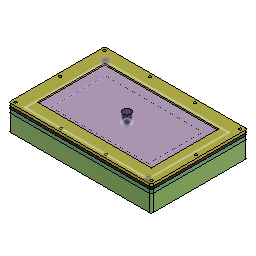
e-ink-photo-frame (Autodesk Fusion 360 design; units mm, degrees)
Autodesk Fusion 360 part; units mm, degrees
(part 1 of 2)
sketch "Sketch1" plane through (0, 0, 0) normal (0, 0, 1) x (1, 0, 0) in component "display-frame"
  line L0 (86, 56) -> (-86, 56)
  line L1 (-86, 56) -> (-86, -56)
  line L2 (-86, -56) -> (86, -56)
  line L3 (86, -56) -> (86, 56)
  line L4 (86, 56) -> (-86, -56) construction
  line L5 (-86, 56) -> (86, -56) construction
  line L6 (15, -65.5) -> (15, -56)
  line L7 (15, -56) -> (-15, -56)
  line L8 (-15, -56) -> (-15, -65.5)
  line L9 (-68, 38) -> (-68, -38)
  line L10 (-68, -38) -> (68, -38)
  line L11 (68, -38) -> (68, 38)
  line L12 (68, 38) -> (-68, 38)
  line L13 (-15, -58.5) -> (15, -58.5)
  line L14 (-15, -59.5) -> (15, -59.5)
  line L15 (80, 49) -> (-80, 49) construction
  line L16 (-80, 49) -> (-80, -46) construction
  line L17 (-80, -46) -> (80, -46) construction
  line L18 (80, -46) -> (80, 49) construction
  line L19 (80, 49) -> (-80, -46) construction
  line L20 (-80, 49) -> (80, -46) construction
  line L21 (-99.5, 68.5) -> (-99.5, -65.5)
  line L22 (-99.5, -65.5) -> (99.5, -65.5)
  line L23 (99.5, -65.5) -> (99.5, 68.5)
  line L24 (99.5, 68.5) -> (-99.5, 68.5)
  point P0 (0, -56)
  point P1 (0, -56)
  point P2 (0, 1.5)
  dimension "d1" = 112
  dimension "d2" = 172
  dimension "d6" = 30
  dimension "d8" = 2.5
  dimension "d30" = 1
  dimension "d86" = -18
  dimension "d91" = 30
  dimension "d93" = 160
  dimension "d94" = 95
  dimension "d96" = 19.5
  dimension "d97" = 9.5
  dimension "d101" = 10
  constraint horizontal L0
  constraint perpendicular L0 L1
  constraint parallel L0 L2
  constraint parallel L1 L3
  constraint coincident L4 origin
  constraint coincident L5 origin
  constraint vertical L6
  constraint horizontal L7
  constraint vertical L8
  constraint coincident L2 L6.end
  constraint midpoint L2 P1
  constraint midpoint L7 P1
  constraint coincident P1 P0
  constraint coincident L8 L13.start
  constraint coincident L6 L13.end
  constraint perpendicular L6 L13
  constraint coincident L8 L14.start
  constraint coincident L6 L14.end
  constraint perpendicular L6 L14
  constraint horizontal L15
  constraint perpendicular L15 L16
  constraint parallel L15 L17
  constraint parallel L16 L18
  constraint coincident L19 P2
  constraint coincident L20 P2
  constraint vertical origin P2
  constraint coincident L8.end L22
  constraint coincident L6.start L22
  measures "d1" distance of L0.end L1.end
  measures "d2" distance of L0.start L0.end
  measures "d6" distance of L6 L8
  measures "d8" distance of L7 L13
  measures "d30" distance of L13 L14
  measures "d91" distance of L14.start L14.end
  measures "d93" distance of L15.start L15.end
  measures "d94" distance of L15.end L16.end
  measures "d97" distance of L2 L22
  measures "d101" distance of L2 L17
extrude "Extrude4" add sketch "Sketch1" along normal blind 0.5 contours L0 L1 L2 L3 L7 | L0 L1 L2 L3 L6 L8 L21 L22 L23 L24 | L2 L6 L7 L8 L13 | L6 L8 L14 L22 makes body 1 in component "display-frame"
extrude "Extrude5" add sketch "Sketch1" along normal blind 3.5 contours L0 L1 L2 L3 L6 L8 L21 L22 L23 L24 | L6 L8 L14 L22 bodies 1 in component "display-frame"
extrude "Extrude6" add sketch "Sketch1" along normal blind 2.5 contours L2 L6 L7 L8 L13 bodies 1 in component "display-frame"
fillet "Fillet3" radius 2.5 1 edges at (0, -58.5, 2.5) on bodies 1 in component "display-frame"
fillet "Fillet4" radius 2.5 4 edges at (-99.5, -65.5, 1.75) (-99.5, 68.5, 1.75) (99.5, 68.5, 1.75) (99.5, -65.5, 1.75) on bodies 1 in component "display-frame"
sketch "Sketch4" plane through (0, 0, 3.5) normal (0, 0, 1) x (-1, 0, 0) in component "display-frame"
  line L0 (-15, 59.5) -> (15, 59.5)
  line L1 (15, 59.5) -> (15, 56)
  line L2 (15, 56) -> (86, 56)
  line L3 (86, 56) -> (86, -56)
  line L4 (86, -56) -> (-86, -56)
  line L5 (-86, -56) -> (-86, 56)
  line L6 (-86, 56) -> (-15, 56)
  line L7 (-15, 56) -> (-15, 59.5)
  arc A0 (-97, 65.5) -> (-99.5, 63) centre (-97, 63) ccw
  line L8 (-99.5, 63) -> (-99.5, -66)
  arc A1 (-99.5, -66) -> (-97, -68.5) centre (-97, -66) ccw
  line L9 (-97, -68.5) -> (97, -68.5)
  arc A2 (97, -68.5) -> (99.5, -66) centre (97, -66) ccw
  line L10 (99.5, -66) -> (99.5, 63)
  arc A3 (99.5, 63) -> (97, 65.5) centre (97, 63) ccw
  line L11 (97, 65.5) -> (-97, 65.5)
  line L12 (99.5, -63.75) -> (-99.5, -63.75) construction
  line L13 (-94.75, -68.5) -> (-94.75, 65.5) construction
  line L14 (99.5, 60.75) -> (-99.5, 60.75) construction
  line L15 (94.75, 65.5) -> (94.75, -68.5) construction
  circle A4 centre (94.75, 60.75) radius 1.75
  circle A5 centre (94.75, -63.75) radius 1.75
  circle A6 centre (31.5833, -63.75) radius 1.75
  circle A7 centre (-31.5833, -63.75) radius 1.75
  circle A8 centre (-94.75, -63.75) radius 1.75
  circle A9 centre (-94.75, 60.75) radius 1.75
  circle A10 centre (-94.75, -1.5) radius 1.75
  circle A11 centre (31.5833, 60.75) radius 1.75
  circle A12 centre (-31.5833, 60.75) radius 1.75
  circle A13 centre (94.75, -1.5) radius 1.75
  dimension "d117" = 9.5
  dimension "d118" = 4.75
  dimension "d119" = 4.75
  dimension "d120" = 4.75
  dimension "d121" = 4.75
  dimension "d122" = 3.5
  dimension "d123" = 189.5
  dimension "d124" = 63.1667
  dimension "d125" = 63.1667
  constraint coincident L10 L12.start
  constraint coincident L8 L12.end
  constraint perpendicular L8 L12
  constraint coincident L9 L13.start
  constraint coincident L11 L13.end
  constraint perpendicular L11 L13
  constraint coincident L10 L14.start
  constraint coincident L8 L14.end
  constraint perpendicular L8 L14
  constraint coincident L11 L15.start
  constraint coincident L9 L15.end
  constraint perpendicular L9 L15
  constraint coincident L15 A4.centre
  constraint coincident L14 A4.centre
  constraint coincident L15 A5.centre
  constraint coincident L12 A5.centre
  constraint coincident L12 A6.centre
  constraint coincident L12 A7.centre
  constraint coincident L13 A8.centre
  constraint coincident L12 A8.centre
  constraint coincident L13 A9.centre
  constraint coincident L14 A9.centre
  constraint midpoint L13 A10.centre
  constraint coincident L14 A11.centre
  constraint coincident L14 A12.centre
  constraint midpoint L15 A13.centre
  constraint equal A5 A6
  constraint equal A6 A7
  constraint equal A7 A8
  constraint equal A8 A10
  constraint equal A9 A10
  constraint equal A9 A12
  constraint equal A11 A12
  constraint equal A4 A11
  constraint equal A4 A13
  constraint vertical A6.centre A11.centre
  constraint vertical A7.centre A12.centre
  measures "d117" distance of L2 L11
  measures "d118" distance of L11 L14
  measures "d119" distance of L10 L15
  measures "d120" distance of L9 L12
  measures "d121" distance of L8 L13
  measures "d122" diameter of A4
  measures "d123" distance of A5.centre A8.centre
  measures "d124" distance of A5.centre A6.centre
  measures "d125" distance of A7.centre A8.centre
extrude "Extrude9" cut sketch "Sketch4" against normal blind 35 contours A4 | A5 | A6 | A7 | A8 | A9 | A10 | A11 | A12 | A13 bodies 1 in component "display-frame"
sketch "Sketch1 (2)" plane through (0, 0, 0) normal (0, 0, -1) x (1, 0, 0) in component "controller-frame"
  circle A0 centre (31.5833, 60.75) radius 1.75
  circle A1 centre (31.5833, -63.75) radius 1.75
  circle A2 centre (-94.75, -1.5) radius 1.75
  circle A3 centre (94.75, -63.75) radius 1.75
  circle A4 centre (-31.5833, 60.75) radius 1.75
  circle A5 centre (94.75, 60.75) radius 1.75
  circle A6 centre (-31.5833, -63.75) radius 1.75
  circle A7 centre (-94.75, -63.75) radius 1.75
  circle A8 centre (94.75, -1.5) radius 1.75
  circle A9 centre (-94.75, 60.75) radius 1.75
  arc A10 (99.5, 63) -> (97, 65.5) centre (97, 63) ccw
  line L0 (97, 65.5) -> (-97, 65.5)
  arc A11 (-97, 65.5) -> (-99.5, 63) centre (-97, 63) ccw
  line L1 (-99.5, 63) -> (-99.5, -66)
  arc A12 (-99.5, -66) -> (-97, -68.5) centre (-97, -66) ccw
  line L2 (-97, -68.5) -> (97, -68.5)
  arc A13 (97, -68.5) -> (99.5, -66) centre (97, -66) ccw
  line L3 (99.5, -66) -> (99.5, 63)
  line L4 (15, 58.5) -> (-15, 58.5)
  line L5 (-15, 58.5) -> (-15, 59.5)
  line L6 (-15, 59.5) -> (15, 59.5)
  line L7 (15, 59.5) -> (15, 58.5)
  line L8 (68, -38) -> (-68, -38)
  line L9 (-68, -38) -> (-68, 38)
  line L10 (-68, 38) -> (68, 38)
  line L11 (68, 38) -> (68, -38)
  line L12 (-86, 56) -> (86, 56)
  line L13 (86, 56) -> (86, -56)
  line L14 (86, -56) -> (-86, -56)
  line L15 (-86, -56) -> (-86, 56)
  line L16 (-68, -38) -> (68, -38)
  line L17 (68, -38) -> (68, 38)
  line L18 (68, 38) -> (-68, 38)
  line L19 (-68, 38) -> (-68, -38)
  line L20 (-15, 56) -> (-15, 58.5)
  line L21 (-15, 58.5) -> (15, 58.5)
  line L22 (15, 58.5) -> (15, 56)
  line L23 (15, 56) -> (-15, 56)
extrude "Extrude2" add sketch "Sketch1 (2)" along normal blind 2.5 separate body contours A10 L0 A11 L1 A12 L2 A13 L3 | L4 L12 L20 L21 L22 L23 | L12 L13 L14 L15 L23 | L8 L9 L10 L11 L16 L17 L18 L19 makes body 2 in component "controller-frame"
sketch "Sketch2" plane through (0, 0, -2.5) normal (0, 0, -1) x (1, 0, 0) in component "controller-frame"
  line L0 (-15, 58.5) -> (-15, 59.5)
  line L1 (15, 59.5) -> (15, 58.5)
  line L2 (15, 58.5) -> (-15, 58.5)
  line L3 (-86, 56) -> (86, 56)
  line L4 (86, 56) -> (86, -56)
  line L5 (86, -56) -> (-86, -56)
  line L6 (-86, -56) -> (-86, 56)
  line L7 (-68, -38) -> (68, -38)
  line L8 (68, -38) -> (68, 38)
  line L9 (68, 38) -> (-68, 38)
  line L10 (-68, 38) -> (-68, -38)
  line L11 (-29, -12) -> (29, -12) construction
  line L12 (29, -12) -> (29, -35) construction
  line L13 (29, -35) -> (-29, -35) construction
  line L14 (-29, -35) -> (-29, -12) construction
  line L15 (-29, -12) -> (29, -35) construction
  line L16 (29, -12) -> (-29, -35) construction
  line L17 (-21.25, 52) -> (21.25, 52) construction
  line L18 (21.25, 52) -> (21.25, 33.5) construction
  line L19 (21.25, 33.5) -> (-21.25, 33.5) construction
  line L20 (-21.25, 33.5) -> (-21.25, 52) construction
  line L21 (-21.25, 52) -> (21.25, 33.5) construction
  line L22 (21.25, 52) -> (-21.25, 33.5) construction
  circle A0 centre (29, -35) radius 1.75
  circle A1 centre (-29, -35) radius 1.75
  circle A2 centre (-29, -12) radius 1.75
  circle A3 centre (29, -12) radius 1.75
  circle A4 centre (29, -35) radius 3
  circle A5 centre (-29, -35) radius 3
  circle A6 centre (-29, -12) radius 3
  circle A7 centre (29, -12) radius 3
  circle A8 centre (18.75, 36) radius 2.5 construction
  circle A9 centre (18.75, 36) radius 1.75
  circle A10 centre (-18.75, 36) radius 2.5 construction
  circle A11 centre (-18.75, 36) radius 1.75
  circle A12 centre (18.75, 49.5) radius 2.5 construction
  circle A13 centre (18.75, 49.5) radius 1
  circle A14 centre (-18.75, 49.5) radius 2.5 construction
  circle A15 centre (-18.75, 49.5) radius 1
  line L23 (-15, 59.5) -> (15, 59.5)
  circle A16 centre (-31.5833, 60.75) radius 1.75
  circle A17 centre (94.75, -1.5) radius 1.75
  circle A18 centre (31.5833, 60.75) radius 1.75
  circle A19 centre (31.5833, -63.75) radius 1.75
  circle A20 centre (-94.75, -1.5) radius 1.75
  circle A21 centre (94.75, -63.75) radius 1.75
  circle A22 centre (-94.75, 60.75) radius 1.75
  circle A23 centre (-94.75, -63.75) radius 1.75
  circle A24 centre (-31.5833, -63.75) radius 1.75
  circle A25 centre (94.75, 60.75) radius 1.75
  line L24 (99.5, -66) -> (99.5, 63)
  arc A26 (99.5, 63) -> (97, 65.5) centre (97, 63) ccw
  line L25 (97, 65.5) -> (-97, 65.5)
  arc A27 (-97, 65.5) -> (-99.5, 63) centre (-97, 63) ccw
  line L26 (-99.5, 63) -> (-99.5, -66)
  arc A28 (-99.5, -66) -> (-97, -68.5) centre (-97, -66) ccw
  line L27 (-97, -68.5) -> (97, -68.5)
  arc A29 (97, -68.5) -> (99.5, -66) centre (97, -66) ccw
  line L28 (-15, 56) -> (-15, 58.5)
  line L29 (-15, 58.5) -> (15, 58.5)
  line L30 (15, 58.5) -> (15, 56)
  line L31 (15, 56) -> (-15, 56)
  point P0 (0, -23.5)
  point P1 (0, 42.75)
  dimension "d134" = 23
  dimension "d135" = 58
  dimension "d136" = 3.5
  dimension "d137" = 6
  dimension "d140" = 5
  dimension "d141" = 3.5
  dimension "d142" = 2
  dimension "d143" = 7.5
  dimension "d234" = 13.5
  dimension "d235" = 37.5
  constraint horizontal L11
  constraint perpendicular L11 L12
  constraint parallel L11 L13
  constraint parallel L12 L14
  constraint coincident L15 P0
  constraint coincident L16 P0
  constraint horizontal L17
  constraint perpendicular L17 L18
  constraint parallel L17 L19
  constraint parallel L18 L20
  constraint coincident L21 P1
  constraint coincident L22 P1
  constraint vertical origin P0
  constraint vertical origin P1
  constraint coincident L12.end L13.start
  constraint coincident L13.end L14.start
  constraint coincident L11.start L14.end
  constraint coincident L11.end L12.start
  constraint equal A2 A3
  constraint equal A1 A2
  constraint equal A0 A1
  constraint concentric A2 A6
  constraint concentric A3 A7
  constraint equal A6 A7
  constraint equal A5 A6
  constraint equal A4 A5
  constraint tangent L7 A4
  constraint concentric A8 A9
  constraint tangent L19 A8
  constraint tangent L18 A8
  constraint concentric A10 A11
  constraint concentric A12 A13
  constraint concentric A14 A15
  constraint equal A13 A15
  constraint equal A9 A11
  constraint equal A10 A14
  constraint equal A12 A14
  constraint equal A8 A12
  constraint tangent L19 A10
  constraint tangent L20 A10
  constraint tangent L17 A12
  constraint tangent L18 A12
  constraint tangent L20 A14
  constraint tangent L17 A14
  measures "d134" distance of L11.end L12.end
  measures "d135" distance of L11.start L11.end
  measures "d136" diameter of A0
  measures "d137" diameter of A4
  measures "d140" diameter of A8
  measures "d141" diameter of A9
  measures "d142" diameter of A13
  measures "d143" distance of L0.end L17
  measures "d234" distance of A8.centre A12.centre
  measures "d235" distance of A8.centre A10.centre
extrude "Extrude4'" add sketch "Sketch2" along normal blind 2.5 contours A5 | A4 | A6 | A7 | A13 | A15 | L24 A26 L25 A27 L26 A28 L27 A29 bodies 2 in component "controller-frame"
extrude "Extrude5'" cut sketch "Sketch2" against normal blind 27 contours A0 | A1 | A2 | A3 | A9 | A11 bodies 2 in component "controller-frame"
fillet "Fillet1" radius 2.5 4 edges at (26.203, 33.9152, -2.5) (-31.797, 33.9152, -2.5) (-31.797, 10.9152, -2.5) (26.203, 10.9152, -2.5) on bodies 2 in component "controller-frame"
fillet "Fillet2" radius 2.5 4 edges at (86, 56, -3.75) (86, -56, -3.75) (-86, -56, -3.75) (-86, 56, -3.75) on bodies 2 in component "controller-frame"
fillet "Fillet3'" radius 2.5 1 edges at (0, -58.5, -2.5) on bodies 2 in component "controller-frame"
sketch "Sketch1 (3)" plane through (0, 0, -5) normal (0, 0, -1) x (1, 0, 0) in component "backing-frame"
  circle A0 centre (-94.75, -63.75) radius 1.75
  line L0 (15, 59.5) -> (15, 56)
  line L1 (15, 56) -> (83.5, 56)
  arc A1 (86, 53.5) -> (83.5, 56) centre (83.5, 53.5) ccw
  line L2 (86, 53.5) -> (86, -53.5)
  arc A2 (83.5, -56) -> (86, -53.5) centre (83.5, -53.5) ccw
  line L3 (83.5, -56) -> (-83.5, -56)
  arc A3 (-86, -53.5) -> (-83.5, -56) centre (-83.5, -53.5) ccw
  line L4 (-86, -53.5) -> (-86, 53.5)
  arc A4 (-83.5, 56) -> (-86, 53.5) centre (-83.5, 53.5) ccw
  line L5 (-83.5, 56) -> (-15, 56)
  line L6 (-15, 56) -> (-15, 59.5)
  line L7 (-15, 59.5) -> (15, 59.5)
  circle A5 centre (-94.75, -1.5) radius 1.75
  circle A6 centre (-31.5833, -63.75) radius 1.75
  circle A7 centre (94.75, 60.75) radius 1.75
  circle A8 centre (31.5833, 60.75) radius 1.75
  circle A9 centre (-31.5833, 60.75) radius 1.75
  circle A10 centre (-94.75, 60.75) radius 1.75
  circle A11 centre (94.75, -63.75) radius 1.75
  circle A12 centre (94.75, -1.5) radius 1.75
  circle A13 centre (31.5833, -63.75) radius 1.75
  arc A14 (97, -68.5) -> (99.5, -66) centre (97, -66) ccw
  line L8 (99.5, -66) -> (99.5, 63)
  arc A15 (99.5, 63) -> (97, 65.5) centre (97, 63) ccw
  line L9 (97, 65.5) -> (-97, 65.5)
  arc A16 (-97, 65.5) -> (-99.5, 63) centre (-97, 63) ccw
  line L10 (-99.5, 63) -> (-99.5, -66)
  arc A17 (-99.5, -66) -> (-97, -68.5) centre (-97, -66) ccw
  line L11 (-97, -68.5) -> (97, -68.5)
  line L12 (15, 58.5) -> (15, 56)
  line L13 (15, 58.5) -> (-15, 58.5)
  line L14 (-15, 56) -> (-15, 58.5)
  line L15 (-15, 56) -> (15, 56)
extrude "Extrude2'" add sketch "Sketch1 (3)" along normal blind 3 separate body contours L0 L6 L7 L13 | L0 L6 L12 L13 L14 L15 | A14 L8 A15 L9 A16 L10 A17 L11 makes body 3 in component "backing-frame"
sketch "Sketch3" plane through (0, 0, -8) normal (0, 0, -1) x (1, 0, 0) in component "backing-frame"
  circle A0 centre (31.5833, -63.75) radius 1.75
  circle A1 centre (94.75, -1.5) radius 1.75
  circle A2 centre (94.75, -63.75) radius 1.75
  circle A3 centre (31.5833, 60.75) radius 1.75
  line L0 (-83.5, 56) -> (83.5, 56)
  arc A4 (86, 53.5) -> (83.5, 56) centre (83.5, 53.5) ccw
  line L1 (86, 53.5) -> (86, -53.5)
  arc A5 (83.5, -56) -> (86, -53.5) centre (83.5, -53.5) ccw
  line L2 (83.5, -56) -> (-83.5, -56)
  line L3 (-86, -53.5) -> (-86, 53.5)
  circle A6 centre (94.75, 60.75) radius 1.75
  line L4 (-97, -68.5) -> (97, -68.5)
  arc A7 (97, -68.5) -> (99.5, -66) centre (97, -66) ccw
  line L5 (99.5, -66) -> (99.5, 63)
  arc A8 (99.5, 63) -> (97, 65.5) centre (97, 63) ccw
  line L6 (97, 65.5) -> (-97, 65.5)
  line L7 (-99.5, 63) -> (-99.5, -66)
  line L8 (94.75, -63.75) -> (83.5, -53.5) construction
  line L9 (94.75, 60.75) -> (83.5, 53.5) construction
  line L10 (94.75, -1.5) -> (86, -1.5) construction
  line L11 (31.5833, -63.75) -> (31.5833, -56) construction
  line L12 (31.5833, 60.75) -> (31.5833, 56) construction
  line L13 (91.65, -3.2898) -> (94.75, -5.0796)
  line L14 (94.75, -5.0796) -> (97.85, -3.2898)
  line L15 (97.85, -3.2898) -> (97.85, 0.2898)
  line L16 (97.85, 0.2898) -> (94.75, 2.0796)
  line L17 (94.75, 2.0796) -> (91.65, 0.2898)
  line L18 (91.65, 0.2898) -> (91.65, -3.2898)
  line L19 (94.75, -5.0796) -> (86, -5.0796)
  line L20 (94.75, 2.0796) -> (86, 2.0796)
  line L21 (81.641, -56) -> (93.9852, -67.2469)
  line L22 (93.9852, -67.2469) -> (97.396, -66.1608)
  line L23 (97.396, -66.1608) -> (98.1608, -62.6639)
  line L24 (98.1608, -62.6639) -> (86, -51.584)
  line L25 (95.5148, -60.2531) -> (92.104, -61.3392)
  line L26 (92.104, -61.3392) -> (91.3392, -64.8361)
  line L27 (86, 51.4231) -> (97.9337, 59.1138)
  line L28 (97.9337, 59.1138) -> (97.7589, 62.6891)
  line L29 (97.7589, 62.6891) -> (94.5752, 64.3253)
  line L30 (94.5752, 64.3253) -> (81.6566, 56)
  line L31 (91.5663, 62.3862) -> (91.7411, 58.8109)
  line L32 (91.7411, 58.8109) -> (94.9248, 57.1747)
  line L33 (29.7935, -60.65) -> (28.0038, -63.75)
  line L34 (28.0038, -63.75) -> (29.7935, -66.85)
  line L35 (29.7935, -66.85) -> (33.3731, -66.85)
  line L36 (33.3731, -66.85) -> (35.1629, -63.75)
  line L37 (35.1629, -63.75) -> (33.3731, -60.65)
  line L38 (33.3731, -60.65) -> (29.7935, -60.65)
  line L39 (28.0038, -63.75) -> (28.0038, -56)
  line L40 (35.1629, -63.75) -> (35.1629, -56)
  line L41 (33.3731, 57.65) -> (35.1629, 60.75)
  line L42 (35.1629, 60.75) -> (33.3731, 63.85)
  line L43 (33.3731, 63.85) -> (29.7935, 63.85)
  line L44 (29.7935, 63.85) -> (28.0038, 60.75)
  line L45 (28.0038, 60.75) -> (29.7935, 57.65)
  line L46 (29.7935, 57.65) -> (33.3731, 57.65)
  line L47 (28.0038, 60.75) -> (28.0038, 56)
  line L48 (35.1629, 60.75) -> (35.1629, 56)
  line L49 (0, -68.5) -> (0, 65.5) construction
  line L50 (-29.7935, 63.85) -> (-28.0038, 60.75)
  line L51 (-33.3731, 63.85) -> (-29.7935, 63.85)
  line L52 (-35.1629, 60.75) -> (-33.3731, 63.85)
  line L53 (-35.1629, 60.75) -> (-35.1629, 56)
  line L54 (-33.3731, 57.65) -> (-35.1629, 60.75)
  line L55 (-29.7935, 57.65) -> (-33.3731, 57.65)
  line L56 (-28.0038, 60.75) -> (-29.7935, 57.65)
  line L57 (-28.0038, 60.75) -> (-28.0038, 56)
  line L58 (-97.9337, 59.1138) -> (-97.7589, 62.6891)
  line L59 (-97.7589, 62.6891) -> (-94.5752, 64.3253)
  line L60 (-94.5752, 64.3253) -> (-81.6566, 56)
  line L61 (-86, 51.4231) -> (-97.9337, 59.1138)
  line L62 (-91.7411, 58.8109) -> (-94.9248, 57.1747)
  line L63 (-91.5663, 62.3862) -> (-91.7411, 58.8109)
  line L64 (-94.75, -5.0796) -> (-86, -5.0796)
  line L65 (-94.75, -5.0796) -> (-97.85, -3.2898)
  line L66 (-97.85, -3.2898) -> (-97.85, 0.2898)
  line L67 (-97.85, 0.2898) -> (-94.75, 2.0796)
  line L68 (-94.75, 2.0796) -> (-86, 2.0796)
  line L69 (-94.75, 2.0796) -> (-91.65, 0.2898)
  line L70 (-91.65, 0.2898) -> (-91.65, -3.2898)
  line L71 (-91.65, -3.2898) -> (-94.75, -5.0796)
  line L72 (-81.641, -56) -> (-93.9852, -67.2469)
  line L73 (-98.1608, -62.6639) -> (-86, -51.584)
  line L74 (-95.5148, -60.2531) -> (-92.104, -61.3392)
  line L75 (-92.104, -61.3392) -> (-91.3392, -64.8361)
  line L76 (-93.9852, -67.2469) -> (-97.396, -66.1608)
  line L77 (-97.396, -66.1608) -> (-98.1608, -62.6639)
  line L78 (-35.1629, -63.75) -> (-35.1629, -56)
  line L79 (-33.3731, -66.85) -> (-35.1629, -63.75)
  line L80 (-29.7935, -66.85) -> (-33.3731, -66.85)
  line L81 (-28.0038, -63.75) -> (-29.7935, -66.85)
  line L82 (-28.0038, -63.75) -> (-28.0038, -56)
  line L83 (-29.7935, -60.65) -> (-28.0038, -63.75)
  line L84 (-33.3731, -60.65) -> (-29.7935, -60.65)
  line L85 (-35.1629, -63.75) -> (-33.3731, -60.65)
  arc A9 (-83.5, 56) -> (-86, 53.5) centre (-83.5, 53.5) ccw
  line L86 (-86, 53.5) -> (-86, -53.5)
  arc A10 (-86, -53.5) -> (-83.5, -56) centre (-83.5, -53.5) ccw
  line L87 (-83.5, -56) -> (83.5, -56)
  arc A11 (83.5, -56) -> (86, -53.5) centre (83.5, -53.5) ccw
  line L88 (86, -53.5) -> (86, 53.5)
  arc A12 (86, 53.5) -> (83.5, 56) centre (83.5, 53.5) ccw
  line L89 (83.5, 56) -> (-83.5, 56)
  circle A13 centre (94.75, 60.75) radius 1.75
  circle A14 centre (-31.5833, -63.75) radius 1.75
  circle A15 centre (31.5833, 60.75) radius 1.75
  circle A16 centre (-94.75, -63.75) radius 1.75
  circle A17 centre (-94.75, -1.5) radius 1.75
  circle A18 centre (-31.5833, 60.75) radius 1.75
  circle A19 centre (-94.75, 60.75) radius 1.75
  circle A20 centre (94.75, -63.75) radius 1.75
  circle A21 centre (94.75, -1.5) radius 1.75
  circle A22 centre (31.5833, -63.75) radius 1.75
  line L90 (97, -68.5) -> (-97, -68.5)
  arc A23 (-99.5, -66) -> (-97, -68.5) centre (-97, -66) ccw
  line L91 (-99.5, -66) -> (-99.5, 63)
  arc A24 (-97, 65.5) -> (-99.5, 63) centre (-97, 63) ccw
  line L92 (-97, 65.5) -> (97, 65.5)
  arc A25 (99.5, 63) -> (97, 65.5) centre (97, 63) ccw
  line L93 (99.5, 63) -> (99.5, -66)
  arc A26 (97, -68.5) -> (99.5, -66) centre (97, -66) ccw
  point P0 (94.75, -1.5)
  point P1 (91.65, -1.5)
  point P2 (94.75, -63.75)
  point P3 (94.75, 60.75)
  point P4 (31.5833, -63.75)
  point P5 (31.5833, -60.65)
  point P6 (31.5833, 60.75)
  point P7 (31.5833, 57.65)
  dimension "d162" = 3.1
  dimension "d163" = 3.1
  dimension "d164" = 3.1
  dimension "d166" = 3.1
  dimension "d167" = 3.1
  constraint coincident P2 A2.centre
  constraint coincident A5.centre L8.end
  constraint coincident P3 A6.centre
  constraint coincident A4.centre L9.end
  constraint coincident P0 A1.centre
  constraint coincident L1 L10.end
  constraint perpendicular L1 L10
  constraint coincident P4 A0.centre
  constraint coincident L2 L11.end
  constraint perpendicular L2 L11
  constraint coincident P6 A3.centre
  constraint coincident L0 L12.end
  constraint perpendicular L0 L12
  constraint midpoint L18 P1
  constraint coincident L10 P1
  constraint coincident L1 L19.end
  constraint perpendicular L1 L19
  constraint coincident L1 L20.end
  constraint perpendicular L1 L20
  constraint coincident L8 L25.end
  constraint coincident L26.end L21
  constraint coincident L25.start L24
  constraint coincident L2 L21.start
  constraint coincident L1 L24.end
  constraint coincident L9 L31.end
  constraint coincident L32.end L27
  constraint coincident L31.start L30
  constraint coincident L1 L27.start
  constraint coincident L0 L30.end
  constraint midpoint L38 P5
  constraint coincident L11 P5
  constraint coincident L2 L39.end
  constraint perpendicular L2 L39
  constraint coincident L2 L40.end
  constraint perpendicular L2 L40
  constraint midpoint L46 P7
  constraint coincident L12 P7
  constraint coincident L0 L47.end
  constraint perpendicular L0 L47
  constraint coincident L0 L48.end
  constraint perpendicular L0 L48
  constraint midpoint L4 L49.start
  constraint midpoint L6 L49.end
  constraint symmetric L13.start L49 L70.end
  constraint symmetric L13.end L49 L64.start
  constraint symmetric L14.end L49 L65.end
  constraint symmetric L15.end L49 L66.end
  constraint symmetric L16.end L49 L67.end
  constraint symmetric L17.end L49 L69.end
  constraint symmetric L19.end L49 L64.end
  constraint symmetric L20.end L49 L68.end
  constraint symmetric L26.end L49 L75.end
  constraint symmetric L21.end L49 L72.end
  constraint symmetric L22.end L49 L76.end
  constraint symmetric L23.end L49 L73.start
  constraint symmetric L25.start L49 L74.start
  constraint symmetric L25.end L49 L74.end
  constraint symmetric L21.start L49 L72.start
  constraint symmetric L24.end L49 L73.end
  constraint symmetric L32.end L49 L62.end
  constraint symmetric L27.end L49 L58.start
  constraint symmetric L28.end L49 L58.end
  constraint symmetric L29.end L49 L59.end
  constraint symmetric L31.start L49 L63.start
  constraint symmetric L31.end L49 L62.start
  constraint symmetric L27.start L49 L61.start
  constraint symmetric L30.end L49 L60.end
  constraint symmetric L33.start L49 L83.start
  constraint symmetric L33.end L49 L81.start
  constraint symmetric L34.end L49 L80.start
  constraint symmetric L35.end L49 L79.start
  constraint symmetric L36.end L49 L78.start
  constraint symmetric L37.end L49 L84.start
  constraint symmetric L39.end L49 L82.end
  constraint symmetric L40.end L49 L78.end
  constraint symmetric L41.start L49 L54.start
  constraint symmetric L41.end L49 L52.start
  constraint symmetric L42.end L49 L51.start
  constraint symmetric L43.end L49 L50.start
  constraint symmetric L44.end L49 L50.end
  constraint symmetric L45.end L49 L55.start
  constraint symmetric L47.end L49 L57.end
  constraint symmetric L48.end L49 L53.end
  measures "d162" distance of P0 L18
  measures "d163" distance of P2 L26
  measures "d164" distance of P3 L32
  measures "d166" distance of P6 L46
  measures "d167" distance of P4 L38
extrude "Extrude5''" add sketch "Sketch3" along normal blind 3.5 contours L0 L3 L60 L61 L62 L63 A9 L86 L89 | L0 L53 L54 L55 L56 L57 L89 | L3 L64 L68 L69 L70 L71 L86 | L0 L41 L45 L46 L47 L48 L89 | L2 L3 L72 L73 L74 L75 L86 A10 L87 | L0 A4 L1 L27 L30 L31 L32 L88 A12 L89 | L2 L78 L82 L83 L84 L85 L87 | L1 L13 L17 L18 L19 L20 L88 | L2 L33 L37 L38 L39 L40 L87 | L1 A5 L2 L21 L24 L25 L26 L87 A11 L88 | L4 A7 L5 A8 L6 L7 L90 A23 L91 A24 L92 A25 L93 A26 bodies 3 in component "backing-frame"
sketch "Sketch9" plane through (0, 0, -11.5) normal (0, 0, -1) x (1, 0, 0) in component "backing-frame"
  line L0 (-93.9852, -67.2469) -> (-97.396, -66.1608) construction
  line L1 (-97.396, -66.1608) -> (-98.1608, -62.6639) construction
  line L2 (-98.1608, -62.6639) -> (-95.5148, -60.2531) construction
  line L3 (-95.5148, -60.2531) -> (-92.104, -61.3392) construction
  line L4 (-92.104, -61.3392) -> (-91.3392, -64.8361) construction
  line L5 (-91.3392, -64.8361) -> (-93.9852, -67.2469) construction
  line L6 (91.3392, -64.8361) -> (92.104, -61.3392) construction
  line L7 (92.104, -61.3392) -> (95.5148, -60.2531) construction
  line L8 (95.5148, -60.2531) -> (98.1608, -62.6639) construction
  line L9 (98.1608, -62.6639) -> (97.396, -66.1608) construction
  line L10 (97.396, -66.1608) -> (93.9852, -67.2469) construction
  line L11 (93.9852, -67.2469) -> (91.3392, -64.8361) construction
  line L12 (94.9248, 57.1747) -> (91.7411, 58.8109) construction
  line L13 (91.7411, 58.8109) -> (91.5663, 62.3862) construction
  line L14 (91.5663, 62.3862) -> (94.5752, 64.3253) construction
  line L15 (94.5752, 64.3253) -> (97.7589, 62.6891) construction
  line L16 (97.7589, 62.6891) -> (97.9337, 59.1138) construction
  line L17 (97.9337, 59.1138) -> (94.9248, 57.1747) construction
  line L18 (-94.5752, 64.3253) -> (-91.5663, 62.3862) construction
  line L19 (-91.5663, 62.3862) -> (-91.7411, 58.8109) construction
  line L20 (-91.7411, 58.8109) -> (-94.9248, 57.1747) construction
  line L21 (-94.9248, 57.1747) -> (-97.9337, 59.1138) construction
  line L22 (-97.9337, 59.1138) -> (-97.7589, 62.6891) construction
  line L23 (-97.7589, 62.6891) -> (-94.5752, 64.3253) construction
  line L24 (91.65, -3.2898) -> (91.65, 0.2898) construction
  line L25 (91.65, 0.2898) -> (94.75, 2.0796) construction
  line L26 (94.75, 2.0796) -> (97.85, 0.2898) construction
  line L27 (97.85, 0.2898) -> (97.85, -3.2898) construction
  line L28 (97.85, -3.2898) -> (94.75, -5.0796) construction
  line L29 (94.75, -5.0796) -> (91.65, -3.2898) construction
  line L30 (33.3731, 57.65) -> (29.7935, 57.65) construction
  line L31 (29.7935, 57.65) -> (28.0038, 60.75) construction
  line L32 (28.0038, 60.75) -> (29.7935, 63.85) construction
  line L33 (29.7935, 63.85) -> (33.3731, 63.85) construction
  line L34 (33.3731, 63.85) -> (35.1629, 60.75) construction
  line L35 (35.1629, 60.75) -> (33.3731, 57.65) construction
  line L36 (-29.7935, 63.85) -> (-28.0038, 60.75) construction
  line L37 (-28.0038, 60.75) -> (-29.7935, 57.65) construction
  line L38 (-29.7935, 57.65) -> (-33.3731, 57.65) construction
  line L39 (-33.3731, 57.65) -> (-35.1629, 60.75) construction
  line L40 (-35.1629, 60.75) -> (-33.3731, 63.85) construction
  line L41 (-33.3731, 63.85) -> (-29.7935, 63.85) construction
  line L42 (29.7935, -60.65) -> (33.3731, -60.65) construction
  line L43 (33.3731, -60.65) -> (35.1629, -63.75) construction
  line L44 (35.1629, -63.75) -> (33.3731, -66.85) construction
  line L45 (33.3731, -66.85) -> (29.7935, -66.85) construction
  line L46 (29.7935, -66.85) -> (28.0038, -63.75) construction
  line L47 (28.0038, -63.75) -> (29.7935, -60.65) construction
  line L48 (-83.5, 56) -> (83.5, 56)
  arc A0 (86, 53.5) -> (83.5, 56) centre (83.5, 53.5) ccw
  line L49 (86, 53.5) -> (86, -53.5)
  arc A1 (83.5, -56) -> (86, -53.5) centre (83.5, -53.5) ccw
  line L50 (83.5, -56) -> (-83.5, -56)
  arc A2 (-86, -53.5) -> (-83.5, -56) centre (-83.5, -53.5) ccw
  line L51 (-86, -53.5) -> (-86, 53.5)
  arc A3 (-83.5, 56) -> (-86, 53.5) centre (-83.5, 53.5) ccw
  line L52 (-91.65, 0.2898) -> (-91.65, -3.2898) construction
  line L53 (-91.65, -3.2898) -> (-94.75, -5.0796) construction
  line L54 (-94.75, -5.0796) -> (-97.85, -3.2898) construction
  line L55 (-97.85, -3.2898) -> (-97.85, 0.2898) construction
  line L56 (-97.85, 0.2898) -> (-94.75, 2.0796) construction
  line L57 (-94.75, 2.0796) -> (-91.65, 0.2898) construction
  line L58 (-33.3731, -66.85) -> (-35.1629, -63.75) construction
  line L59 (-35.1629, -63.75) -> (-33.3731, -60.65) construction
  line L60 (-33.3731, -60.65) -> (-29.7935, -60.65) construction
  line L61 (-29.7935, -60.65) -> (-28.0038, -63.75) construction
  line L62 (-28.0038, -63.75) -> (-29.7935, -66.85) construction
  line L63 (-29.7935, -66.85) -> (-33.3731, -66.85) construction
  arc A4 (-99.5, -66) -> (-97, -68.5) centre (-97, -66) ccw
  line L64 (-97, -68.5) -> (97, -68.5)
  arc A5 (97, -68.5) -> (99.5, -66) centre (97, -66) ccw
  line L65 (99.5, -66) -> (99.5, 63)
  arc A6 (99.5, 63) -> (97, 65.5) centre (97, 63) ccw
  line L66 (97, 65.5) -> (-97, 65.5)
  arc A7 (-97, 65.5) -> (-99.5, 63) centre (-97, 63) ccw
  line L67 (-99.5, 63) -> (-99.5, -66)
  line L68 (29.7935, -60.65) -> (-29.7935, -60.65) construction
  line L69 (-29.7935, -60.65) -> (-29.7935, -66.85) construction
  line L70 (-29.7935, -66.85) -> (29.7935, -66.85) construction
  line L71 (29.7935, -66.85) -> (29.7935, -60.65) construction
  dimension "d192" = 4
  text T0 "INSERT BOLTS" font "Courier New" height 4 bold align centre bottom in box 59.5871 x 6.2 at (29.7935, -60.65) x (-1, 0) y (0, -1) spacing 1 kerned
  constraint coincident L60.end
  constraint coincident L45.end
extrude "Extrude6'" cut sketch "Sketch9" against normal blind 0.75 text T0 bodies 3 in component "backing-frame"
extrude "Extrude7" add sketch "Sketch9" along normal blind 13.8 bodies 3 in component "backing-frame"
sketch "Sketch10" plane through (0, 0, -11.5) normal (0, 0, -1) x (1, 0, 0) in component "backing-frame"
  circle A0 centre (94.75, 60.75) radius 1.75
  circle A1 centre (31.5833, 60.75) radius 1.75
  circle A2 centre (-31.5833, 60.75) radius 1.75
  circle A3 centre (-94.75, 60.75) radius 1.75
  circle A4 centre (-94.75, -1.5) radius 1.75
  circle A5 centre (-94.75, -63.75) radius 1.75
  circle A6 centre (-31.5833, -63.75) radius 1.75
  circle A7 centre (31.5833, -63.75) radius 1.75
  circle A8 centre (94.75, -63.75) radius 1.75
  circle A9 centre (94.75, -1.5) radius 1.75
extrude "Extrude8" cut sketch "Sketch10" along normal blind 10 bodies 3 in component "backing-frame"
sketch "Sketch1 (4)" plane through (0, 0, 3.5) normal (0, 0, 1) x (-1, 0, 0) in component "glass-frame"
  circle A0 centre (-31.5833, 60.75) radius 1.75
  circle A1 centre (-31.5833, -63.75) radius 1.75
  circle A2 centre (94.75, -1.5) radius 1.75
  circle A3 centre (-94.75, -63.75) radius 1.75
  circle A4 centre (31.5833, 60.75) radius 1.75
  circle A5 centre (-94.75, 60.75) radius 1.75
  circle A6 centre (31.5833, -63.75) radius 1.75
  circle A7 centre (94.75, -63.75) radius 1.75
  circle A8 centre (-94.75, -1.5) radius 1.75
  circle A9 centre (94.75, 60.75) radius 1.75
  line L0 (-15, 59.5) -> (15, 59.5) construction
  line L1 (15, 59.5) -> (15, 56) construction
  line L2 (15, 56) -> (86, 56) construction
  line L3 (86, 56) -> (86, -56) construction
  line L4 (86, -56) -> (-86, -56) construction
  line L5 (-86, -56) -> (-86, 56) construction
  line L6 (-86, 56) -> (-15, 56) construction
  line L7 (-15, 56) -> (-15, 59.5) construction
  arc A10 (-97, 65.5) -> (-99.5, 63) centre (-97, 63) ccw
  line L8 (-99.5, 63) -> (-99.5, -66)
  arc A11 (-99.5, -66) -> (-97, -68.5) centre (-97, -66) ccw
  line L9 (-97, -68.5) -> (97, -68.5)
  arc A12 (97, -68.5) -> (99.5, -66) centre (97, -66) ccw
  line L10 (99.5, -66) -> (99.5, 63)
  arc A13 (99.5, 63) -> (97, 65.5) centre (97, 63) ccw
  line L11 (97, 65.5) -> (-97, 65.5)
  line L12 (89, -57) -> (-89, -57)
  line L13 (-89, -57) -> (-89, 56)
  line L14 (-89, 56) -> (89, 56)
  line L15 (89, 56) -> (89, -57)
  point P0 (0, -56)
  point P1 (0, -57)
  dimension "d236" = 9.5
  dimension "d240" = 178
  dimension "d241" = 113
  constraint horizontal L12
  constraint vertical L13
  constraint horizontal L14
  constraint vertical L15
  constraint coincident L2.end L14
  constraint midpoint L4 P0
  constraint midpoint L12 P1
  constraint vertical P0 P1
  measures "d236" distance of L11 L14
  measures "d240" distance of L12.start L12.end
  measures "d241" distance of L12.end L13.end
extrude "Extrude1" add sketch "Sketch1 (4)" along normal blind 1.65 separate body makes body 4 in component "glass-frame"
sketch "Sketch2 (2)" plane through (0, 0, 5.15) normal (0, 0, 1) x (-1, 0, 0) in component "glass-frame"
  line L0 (-89, 56) -> (89, 56)
  line L1 (89, 56) -> (89, -57)
  line L2 (89, -57) -> (-89, -57)
  line L3 (-89, -57) -> (-89, 56)
  circle A0 centre (-94.75, -1.5) radius 1.75
  circle A1 centre (31.5833, -63.75) radius 1.75
  circle A2 centre (94.75, 60.75) radius 1.75
  circle A3 centre (-31.5833, 60.75) radius 1.75
  circle A4 centre (31.5833, 60.75) radius 1.75
  circle A5 centre (94.75, -63.75) radius 1.75
  circle A6 centre (-94.75, -63.75) radius 1.75
  circle A7 centre (-31.5833, -63.75) radius 1.75
  circle A8 centre (94.75, -1.5) radius 1.75
  circle A9 centre (-94.75, 60.75) radius 1.75
  line L4 (97, 65.5) -> (-97, 65.5)
  arc A10 (-97, 65.5) -> (-99.5, 63) centre (-97, 63) ccw
  line L5 (-99.5, 63) -> (-99.5, -66)
  arc A11 (-99.5, -66) -> (-97, -68.5) centre (-97, -66) ccw
  line L6 (-97, -68.5) -> (97, -68.5)
  arc A12 (97, -68.5) -> (99.5, -66) centre (97, -66) ccw
  line L7 (99.5, -66) -> (99.5, 63)
  arc A13 (99.5, 63) -> (97, 65.5) centre (97, 63) ccw
  line L8 (80, -49) -> (80, 46)
  line L9 (-80, -49) -> (80, -49)
  line L10 (-80, 46) -> (-80, -49)
  line L11 (80, 46) -> (-80, 46)
  line L12 (99.5, -66) -> (99.5, 63)
  arc A14 (97, -68.5) -> (99.5, -66) centre (97, -66) ccw
  line L13 (-97, -68.5) -> (97, -68.5)
  arc A15 (-99.5, -66) -> (-97, -68.5) centre (-97, -66) ccw
  line L14 (-99.5, 63) -> (-99.5, -66)
  arc A16 (-97, 65.5) -> (-99.5, 63) centre (-97, 63) ccw
  line L15 (97, 65.5) -> (-97, 65.5)
  arc A17 (99.5, 63) -> (97, 65.5) centre (97, 63) ccw
  line L16 (-79.5, 45.5) -> (-79.5, -48.5)
  line L17 (-79.5, -48.5) -> (79.5, -48.5)
  line L18 (79.5, -48.5) -> (79.5, 45.5)
  line L19 (79.5, 45.5) -> (-79.5, 45.5)
  line L20 (83, 49) -> (-83, 49)
  line L21 (-83, 49) -> (-83, -52)
  line L22 (-83, -52) -> (83, -52)
  line L23 (83, -52) -> (83, 49)
  dimension "d203" = -0.5
  dimension "d239" = 3
extrude "Extrude2''" add sketch "Sketch2 (2)" along normal blind 2 contours L0 L1 L2 L3 | L4 A10 L5 A11 L6 A12 L7 A13 L12 A14 L13 A15 L14 A16 L15 A17 | L8 L9 L10 L11 | L20 L21 L22 L23 bodies 4 in component "glass-frame"
sketch "Sketch18" plane through (0, 0, -25.3) normal (0, 0, -1) x (1, 0, 0) in component "backing-frame"
  arc A0 (86, 53.5) -> (83.5, 56) centre (83.5, 53.5) ccw
  line L0 (86, 53.5) -> (86, -53.5)
  arc A1 (83.5, -56) -> (86, -53.5) centre (83.5, -53.5) ccw
  line L1 (83.5, -56) -> (-83.5, -56)
  arc A2 (-86, -53.5) -> (-83.5, -56) centre (-83.5, -53.5) ccw
  line L2 (-86, -53.5) -> (-86, 53.5)
  arc A3 (-83.5, 56) -> (-86, 53.5) centre (-83.5, 53.5) ccw
  line L3 (-83.5, 56) -> (83.5, 56)
  line L4 (-99.5, 63) -> (-99.5, -66)
  arc A4 (-99.5, -66) -> (-97, -68.5) centre (-97, -66) ccw
  line L5 (-97, -68.5) -> (97, -68.5)
  arc A5 (97, -68.5) -> (99.5, -66) centre (97, -66) ccw
  line L6 (99.5, -66) -> (99.5, 63)
  arc A6 (99.5, 63) -> (97, 65.5) centre (97, 63) ccw
  line L7 (97, 65.5) -> (-97, 65.5)
  arc A7 (-97, 65.5) -> (-99.5, 63) centre (-97, 63) ccw
  line L8 (0, 65.5) -> (0, -68.5) construction
  circle A8 centre (-66.3333, -58.5) radius 10
  circle A9 centre (-66.3333, -58.5) radius 5
  circle A10 centre (66.3333, -58.5) radius 5
  circle A11 centre (66.3333, -58.5) radius 10
  dimension "d253" = 10
  dimension "d254" = 20
  dimension "d255" = 99.5
  dimension "d256" = 33.1667
  constraint midpoint L7 L8.start
  constraint midpoint L5 L8.end
  constraint concentric A8 A9
  constraint tangent L5 A8
  constraint symmetric L8 A8 A11
  constraint symmetric L8 A9 A10
  measures "d253" diameter of A9
  measures "d254" diameter of A8
  measures "d255" distance of L4 L8
  measures "d256" distance of L4 A8.centre
extrude "Extrude10" add sketch "Sketch18" against normal blind 20.3 contours L1 A10 A11 | L1 A10 | L1 A8 A9 | L1 A9 picked at (58.9692, -54.6415) picked at (66.5817, -54.7736) picked at (-73.6974, -54.6415) picked at (-65.8421, -54.8291) bodies 3 in component "backing-frame"
extrude "Extrude11" cut sketch "Sketch18" against normal blind 15.3 contours L1 A10 | L1 A10 | L1 A9 | L1 A9 bodies 3 in component "backing-frame"
sketch "Sketch19" plane through (0, 0, -25.3) normal (0, 0, -1) x (1, 0, 0) in component "backing-frame"
  circle A0 centre (66.3333, -58.5) radius 5
  circle A1 centre (-66.3333, -58.5) radius 5
  arc A2 (86, 53.5) -> (83.5, 56) centre (83.5, 53.5) ccw
  line L0 (86, 53.5) -> (86, -53.5)
  arc A3 (83.5, -56) -> (86, -53.5) centre (83.5, -53.5) ccw
  line L1 (83.5, -56) -> (76.0158, -56)
  arc A4 (76.0158, -56) -> (56.6509, -56) centre (66.3333, -58.5) ccw
  line L2 (56.6509, -56) -> (-56.6509, -56)
  arc A5 (-56.6509, -56) -> (-76.0158, -56) centre (-66.3333, -58.5) ccw
  line L3 (-76.0158, -56) -> (-83.5, -56)
  arc A6 (-86, -53.5) -> (-83.5, -56) centre (-83.5, -53.5) ccw
  line L4 (-86, -53.5) -> (-86, 53.5)
  arc A7 (-83.5, 56) -> (-86, 53.5) centre (-83.5, 53.5) ccw
  line L5 (-83.5, 56) -> (83.5, 56)
  line L6 (-99.5, 63) -> (-99.5, -66)
  arc A8 (-99.5, -66) -> (-97, -68.5) centre (-97, -66) ccw
  line L7 (-97, -68.5) -> (97, -68.5)
  arc A9 (97, -68.5) -> (99.5, -66) centre (97, -66) ccw
  line L8 (99.5, -66) -> (99.5, 63)
  arc A10 (99.5, 63) -> (97, 65.5) centre (97, 63) ccw
  line L9 (97, 65.5) -> (-97, 65.5)
  arc A11 (-97, 65.5) -> (-99.5, 63) centre (-97, 63) ccw
  arc A12 (90, 53.5) -> (83.5, 60) centre (83.5, 53.5) ccw
  line L10 (-83.5, 60) -> (83.5, 60)
  arc A13 (-83.5, 60) -> (-90, 53.5) centre (-83.5, 53.5) ccw
  line L11 (-90, -53.5) -> (-90, 53.5)
  arc A14 (-90, -53.5) -> (-83.5, -60) centre (-83.5, -53.5) ccw
  line L12 (-72.1428, -60) -> (-83.5, -60)
  arc A15 (-60.5239, -60) -> (-72.1428, -60) centre (-66.3333, -58.5) ccw
  line L13 (60.5239, -60) -> (-60.5239, -60)
  arc A16 (72.1428, -60) -> (60.5239, -60) centre (66.3333, -58.5) ccw
  line L14 (83.5, -60) -> (72.1428, -60)
  arc A17 (83.5, -60) -> (90, -53.5) centre (83.5, -53.5) ccw
  line L15 (90, 53.5) -> (90, -53.5)
  dimension "d261" = -4
extrude "Extrude12" add sketch "Sketch19" along normal blind 3 contours L6 A8 L7 A9 L8 A10 L9 A11 bodies 3 in component "backing-frame"
sketch "Sketch20" plane through (0, 0, -28.3) normal (0, 0, -1) x (1, 0, 0) in component "backing-frame"
  circle A0 centre (-66.3333, -58.5) radius 5
  circle A1 centre (66.3333, -58.5) radius 5
  arc A2 (-83.5, 60) -> (-90, 53.5) centre (-83.5, 53.5) ccw
  line L0 (-83.5, 60) -> (83.5, 60)
  arc A3 (90, 53.5) -> (83.5, 60) centre (83.5, 53.5) ccw
  line L1 (90, 53.5) -> (90, -53.5)
  arc A4 (83.5, -60) -> (90, -53.5) centre (83.5, -53.5) ccw
  line L2 (83.5, -60) -> (72.1428, -60)
  arc A5 (72.1428, -60) -> (60.5239, -60) centre (66.3333, -58.5) ccw
  line L3 (60.5239, -60) -> (-60.5239, -60)
  arc A6 (-60.5239, -60) -> (-72.1428, -60) centre (-66.3333, -58.5) ccw
  line L4 (-72.1428, -60) -> (-83.5, -60)
  arc A7 (-90, -53.5) -> (-83.5, -60) centre (-83.5, -53.5) ccw
  line L5 (-90, -53.5) -> (-90, 53.5)
  arc A8 (-97, 65.5) -> (-99.5, 63) centre (-97, 63) ccw
  line L6 (-99.5, 63) -> (-99.5, -66)
  arc A9 (-99.5, -66) -> (-97, -68.5) centre (-97, -66) ccw
  line L7 (-97, -68.5) -> (97, -68.5)
  arc A10 (97, -68.5) -> (99.5, -66) centre (97, -66) ccw
  line L8 (99.5, -66) -> (99.5, 63)
  arc A11 (99.5, 63) -> (97, 65.5) centre (97, 63) ccw
  line L9 (97, 65.5) -> (-97, 65.5)
  line L10 (-90, 53.5) -> (-90, -53.5)
  arc A12 (-90, -53.5) -> (-83.5, -60) centre (-83.5, -53.5) ccw
  line L11 (-83.5, -60) -> (-72.1428, -60)
  arc A13 (-60.5239, -60) -> (-72.1428, -60) centre (-66.3333, -58.5) ccw
  line L12 (-60.5239, -60) -> (60.5239, -60)
  arc A14 (72.1428, -60) -> (60.5239, -60) centre (66.3333, -58.5) ccw
  line L13 (72.1428, -60) -> (83.5, -60)
  arc A15 (83.5, -60) -> (90, -53.5) centre (83.5, -53.5) ccw
  line L14 (90, -53.5) -> (90, 53.5)
  arc A16 (90, 53.5) -> (83.5, 60) centre (83.5, 53.5) ccw
  line L15 (83.5, 60) -> (-83.5, 60)
  arc A17 (-83.5, 60) -> (-90, 53.5) centre (-83.5, 53.5) ccw
  arc A18 (86, 53.5) -> (83.5, 56) centre (83.5, 53.5) ccw
  line L16 (86, 53.5) -> (86, -53.5)
  arc A19 (83.5, -56) -> (86, -53.5) centre (83.5, -53.5) ccw
  line L17 (83.5, -56) -> (76.0158, -56)
  arc A20 (76.0158, -56) -> (56.6509, -56) centre (66.3333, -58.5) ccw
  line L18 (56.6509, -56) -> (-56.6509, -56)
  arc A21 (-56.6509, -56) -> (-76.0158, -56) centre (-66.3333, -58.5) ccw
  line L19 (-76.0158, -56) -> (-83.5, -56)
  arc A22 (-86, -53.5) -> (-83.5, -56) centre (-83.5, -53.5) ccw
  line L20 (-86, -53.5) -> (-86, 53.5)
  arc A23 (-83.5, 56) -> (-86, 53.5) centre (-83.5, 53.5) ccw
  line L21 (-83.5, 56) -> (83.5, 56)
  circle A24 centre (0, 61.5) radius 2.75
  circle A25 centre (0, 61.5) radius 1.5
  line L22 (-90, 0) -> (90, 0) construction
  circle A26 centre (-89.1569, 59.1569) radius 2.75
  circle A27 centre (-89.1569, 59.1569) radius 1.5
  circle A28 centre (89.1569, 59.1569) radius 2.75
  circle A29 centre (89.1569, 59.1569) radius 1.5
  circle A30 centre (-89.1569, -59.1569) radius 1.5
  circle A31 centre (-89.1569, -59.1569) radius 2.75
  circle A32 centre (0, -61.5) radius 1.5
  circle A33 centre (0, -61.5) radius 2.75
  circle A34 centre (89.1569, -59.1569) radius 1.5
  circle A35 centre (89.1569, -59.1569) radius 2.75
  point P0 (0, 60)
  point P1 (-88.0962, 58.0962)
  point P2 (88.0962, 58.0962)
  dimension "d264" = 5.5
  dimension "d265" = 3
  constraint concentric A24 A25
  constraint tangent L0 A25
  constraint midpoint L15 P0
  constraint coincident A25 P0
  constraint midpoint A17 P1
  constraint midpoint A16 P2
  constraint midpoint L10 L22.start
  constraint midpoint L14 L22.end
  constraint concentric A26 A27
  constraint concentric A28 A29
  constraint equal A26 A28
  constraint equal A24 A28
  constraint equal A27 A29
  constraint equal A25 A29
  constraint tangent A2 A27
  constraint tangent A16 A29
  constraint coincident P1 A27
  constraint coincident P2 A29
  constraint symmetric A24 L22 A33
  constraint symmetric A25 L22 A32
  constraint symmetric L22 A26 A31
  constraint symmetric L22 A27 A30
  constraint symmetric L22 A28 A35
  constraint symmetric L22 A29 A34
  measures "d264" diameter of A24
  measures "d265" diameter of A25
extrude "Extrude13" cut sketch "Sketch20" against normal blind 3 contours A2 A17 A26 | L0 L15 A24 | A3 A16 A28 | A7 A12 A31 | A4 A15 A35 | L3 L12 A33 picked at (-89.406, 57.0616) picked at (-2.0311, 60.3623) picked at (87.0587, 59.394) picked at (-89.406, -57.0616) picked at (87.0587, -59.394) picked at (-2.0311, -60.3623) bodies 3 in component "backing-frame"
extrude "Extrude14" cut sketch "Sketch20" against normal blind 15 contours A27 | A25 | A29 | A30 | A34 | A32 bodies 3 in component "backing-frame"
sketch "Sketch1 (5)" plane through (0, 0, -25.3) normal (0, 0, -1) x (1, 0, 0) in component "backing"
  circle A0 centre (89.1569, 59.1569) radius 1.5
  circle A1 centre (-89.1569, -59.1569) radius 1.5
  circle A2 centre (89.1569, -59.1569) radius 1.5
  circle A3 centre (0, 61.5) radius 1.5
  circle A4 centre (-89.1569, 59.1569) radius 1.5
  circle A5 centre (0, -61.5) radius 1.5
  arc A6 (89.3116, 56.4112) -> (86.4112, 59.3116) centre (89.1569, 59.1569) ccw
  arc A7 (86.4112, 59.3116) -> (83.5, 60) centre (83.5, 53.5) ccw
  line L0 (83.5, 60) -> (2.3049, 60)
  arc A8 (2.3049, 60) -> (-2.3049, 60) centre (0, 61.5) ccw
  line L1 (-2.3049, 60) -> (-83.5, 60)
  arc A9 (-83.5, 60) -> (-86.4112, 59.3116) centre (-83.5, 53.5) ccw
  arc A10 (-86.4112, 59.3116) -> (-89.3116, 56.4112) centre (-89.1569, 59.1569) ccw
  arc A11 (-89.3116, 56.4112) -> (-90, 53.5) centre (-83.5, 53.5) ccw
  line L2 (-90, 53.5) -> (-90, -53.5)
  arc A12 (-90, -53.5) -> (-89.3116, -56.4112) centre (-83.5, -53.5) ccw
  arc A13 (-89.3116, -56.4112) -> (-86.4112, -59.3116) centre (-89.1569, -59.1569) ccw
  arc A14 (-86.4112, -59.3116) -> (-83.5, -60) centre (-83.5, -53.5) ccw
  line L3 (-83.5, -60) -> (-72.1428, -60)
  arc A15 (-60.5239, -60) -> (-72.1428, -60) centre (-66.3333, -58.5) ccw
  line L4 (-60.5239, -60) -> (-2.3049, -60)
  arc A16 (-2.3049, -60) -> (2.3049, -60) centre (0, -61.5) ccw
  line L5 (2.3049, -60) -> (60.5239, -60)
  arc A17 (72.1428, -60) -> (60.5239, -60) centre (66.3333, -58.5) ccw
  line L6 (72.1428, -60) -> (83.5, -60)
  arc A18 (83.5, -60) -> (86.4112, -59.3116) centre (83.5, -53.5) ccw
  arc A19 (86.4112, -59.3116) -> (89.3116, -56.4112) centre (89.1569, -59.1569) ccw
  arc A20 (89.3116, -56.4112) -> (90, -53.5) centre (83.5, -53.5) ccw
  line L7 (90, -53.5) -> (90, 53.5)
  arc A21 (90, 53.5) -> (89.3116, 56.4112) centre (83.5, 53.5) ccw
extrude "Extrude1'" add sketch "Sketch1 (5)" along normal blind 2 separate body makes body 5 in component "backing"
sketch "Sketch1 (6)" plane through (0, 0, 0) normal (0, 0, 1) x (1, 0, 0) in component "bolt-test"
  circle A0 centre (0, 0) radius 5.6
  line L0 (3.1, 1.7898) -> (0, 3.5796)
  line L1 (0, 3.5796) -> (-3.1, 1.7898)
  line L2 (-3.1, 1.7898) -> (-3.1, -1.7898)
  line L3 (-3.1, -1.7898) -> (0, -3.5796)
  line L4 (0, -3.5796) -> (3.1, -1.7898)
  line L5 (3.1, -1.7898) -> (3.1, 1.7898)
  circle A1 centre (0, 0) radius 1.75
  dimension "d242" = 3.1
  dimension "d243" = 11.2
  dimension "d244" = 3.5
  constraint coincident A0.centre A1.centre
  constraint vertical A0.centre L0.end
  measures "d242" distance of A0.centre L5
  measures "d243" diameter of A0
  measures "d244" diameter of A1
extrude "Extrude1''" add sketch "Sketch1 (6)" along normal blind 3 separate body contours A0 | L0 L1 L2 L3 L4 L5 makes body 6 in component "bolt-test"
extrude "Extrude2'''" add sketch "Sketch1 (6)" along normal blind 6.5 contours A0 bodies 6 in component "bolt-test"
sketch "Sketch2 (3)" plane through (0, 0, 6.5) normal (0, 0, 1) x (-1, 0, 0) in component "bolt-test"
  line L0 (-3.1, -1.7898) -> (-3.1, 1.7898)
  line L1 (-3.1, 1.7898) -> (0, 3.5796)
  line L2 (0, 3.5796) -> (3.1, 1.7898)
  line L3 (3.1, 1.7898) -> (3.1, -1.7898)
  line L4 (3.1, -1.7898) -> (0, -3.5796)
  line L5 (0, -3.5796) -> (-3.1, -1.7898)
  circle A0 centre (0, 0) radius 5.6
  circle A1 centre (0, 0) radius 1.75
  circle A2 centre (0, 0) radius 5.6
extrude "Extrude3" add sketch "Sketch2 (3)" along normal blind 3 contours L0 L1 L2 L3 L4 L5 | A0 A2 bodies 6 in component "bolt-test"
sketch "Sketch3 (2)" plane through (0, 0, 9.5) normal (0, 0, 1) x (-1, 0, 0) in component "bolt-test"
  circle A0 centre (0, 0) radius 1.75
  circle A1 centre (0, 0) radius 5.6
  circle A2 centre (0, 0) radius 5.6
extrude "Extrude4''" add sketch "Sketch3 (2)" along normal blind 3 contours A0 | A1 A2 bodies 6 in component "bolt-test"